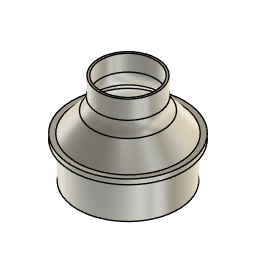
universal_dust_extraction_adapter_bms_v13 (Autodesk Fusion 360 design; units mm, degrees)
Autodesk Fusion 360 part; units mm, degrees
sketch "Sketch1" plane through (0, 0, 0) normal (0, 0, 1) x (1, 0, 0)
  circle A0 centre (0, 0) radius 50
  circle A1 centre (0, 0) radius 47
  dimension "d1" = 100
  dimension "d9" = -3
  constraint coincident A0.centre A1.centre
  measures "d1" diameter of A0
ref_plane "WorkPlane1" through (0, 0, 41) normal (0, 0, 1) x (1, 0, 0)
sketch "Sketch2" plane through (0, 0, 41) normal (0, 0, 1) x (1, 0, 0)
  circle A0 centre (0, 0) radius 51
  circle A1 centre (0, 0) radius 48
  dimension "d4" = 102
  dimension "d10" = -3
  constraint coincident A0.centre A1.centre
  measures "d4" diameter of A0
ref_plane "WorkPlane2" through (0, 0, 66) normal (0, 0, 1) x (1, 0, 0)
sketch "Sketch5" plane through (0, 0, 66) normal (0, 0, 1) x (1, 0, 0)
  circle A0 centre (0, 0) radius 29.75
  circle A1 centre (0, 0) radius 27.75
  dimension "d22" = 59.5
  dimension "d23" = -2
  constraint coincident A0.centre A1.centre
  measures "d22" diameter of A0
ref_plane "WorkPlane3" through (0, 0, 91) normal (0, 0, 1) x (1, 0, 0)
sketch "Sketch6" plane through (0, 0, 91) normal (0, 0, 1) x (1, 0, 0)
  circle A0 centre (0, 0) radius 29
  circle A1 centre (0, 0) radius 27
  dimension "d25" = 58
  dimension "d26" = -2
  constraint coincident A0.centre A1.centre
  measures "d25" diameter of A0
sketch "Sketch7" plane through (0, 0, 0) normal (0, 1, 0) x (1, 0, 0)
  line L0 (-47, 0) -> (47, 0)
  line L1 (-50, 0) -> (50, 0)
  line L2 (-51, -41) -> (51, -41)
  line L3 (-48, -41) -> (48, -41)
  line L4 (-27.75, -66) -> (27.75, -66)
  line L5 (-29.75, -66) -> (29.75, -66)
  line L6 (-27, -91) -> (27, -91)
  line L7 (-29, -91) -> (29, -91)
  line L8 (-50, 0) -> (-51, -41)
  line L9 (-47, 0) -> (-48, -41)
  line L10 (-48, -41) -> (-27.75, -66)
  line L11 (-51, -41) -> (-29.75, -66)
  line L12 (-29.75, -66) -> (-29, -91)
  line L13 (-27.75, -66) -> (-27, -91)
  line L14 (-51, -41) -> (-56, -41)
  line L15 (-56, -41) -> (-56, -36)
  line L16 (-56, -36) -> (-51, -36)
  line L17 (-51, -36) -> (-51, -41) construction
  line L18 (-51, -36) -> (-50.878, -36)
  line L19 (0, 0) -> (0, -91) construction
  dimension "d27" = 5
  dimension "d28" = 5
  constraint coincident L1.start L8.start
  constraint coincident L2.start L8.end
  constraint coincident L0.start L9.start
  constraint coincident L3.start L9.end
  constraint coincident L4.start L10.end
  constraint coincident L5.start L11.end
  constraint coincident L7.start L12.end
  constraint coincident L6.start L13.end
  constraint horizontal L14
  constraint vertical L15
  constraint horizontal L16
  constraint vertical L17
  constraint coincident L8 L18.end
  constraint perpendicular L17 L18
  constraint coincident L19.start origin
  constraint midpoint L7 L19.end
  measures "d27" distance of L2.start L14.end
  measures "d28" distance of L2.start L16.end
revolve "Revolve2" add sketch "Sketch7" angle 360 about axis through (0, 0, 0) along (0, 0, 1)
fillet "Fillet4" radius 40 1 edges at (-44.7517, 17.3575, 41)
fillet "Fillet5" radius 25 1 edges at (-25.8721, 10.0348, 66)
fillet "Fillet6" radius 20 1 edges at (-27.7367, 10.7581, 66)
